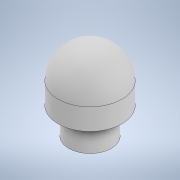
# Autodesk Inventor part: head
Saved by Autodesk Inventor 2022 (Build 260153000, 153)
## iProperties
Created: 2023-01-18
Part Number: head
Material: Generic
Document SubType Name: Modeling
Designer: zhong
Density: 1 g/cm^3
Appearance: Default
Author: zhong
Autodesk Inventor part; units mm, degrees
ref_plane "YZ Plane" through (0, 0, 0) normal (1, 0, 0) x (0, 1, 0)
ref_plane "XZ Plane" through (0, 0, 0) normal (0, 1, 0) x (-1, 0, 0)
ref_plane "XY Plane" through (0, 0, 0) normal (0, 0, 1) x (1, 0, 0)
sketch "Sketch1" plane through (0, 0, 0) normal (1, 0, 0) x (0, 1, 0)
  line L0 (0, 6) -> (4, 6)
  line L1 (0, -6) -> (4, -6)
  arc A0 (4, -6) -> (4, 6) centre (4, 0) ccw
  line L2 (0, 6) -> (0, 4)
  line L3 (0, 4) -> (-5, 4)
  line L4 (0, -6) -> (0, -4)
  line L5 (0, -4) -> (-5, -4)
  arc A1 (4, -4) -> (4, 4) centre (4, 0) ccw
  line L6 (2, 4) -> (4, 4)
  line L7 (2, -4) -> (4, -4)
  line L8 (2, -4) -> (2, -3)
  line L9 (2, -3) -> (-5, -3)
  line L10 (2, 4) -> (2, 3)
  line L11 (2, 3) -> (-5, 3)
  line L12 (-5, 4) -> (-5, 3)
  line L13 (-5, -3) -> (-5, -4)
  line L14 (-5, 0) -> (10, 0)
  point P0 (0, 0)
  point P1 (8, 0)
  dimension "d0" = 4
  dimension "d1" = 2
  dimension "d2" = 5
  dimension "d3" = 2
  dimension "d4" = 1
  dimension "d5" = 1
  constraints: 30 end point, 5 perpendicular, 5 point on circle, 5 vertical, 2 centre point, 2 horizontal, 2 tangent, 1 coincident
  measures "d0" distance of L0.start L0.end
  measures "d1" distance of L0.start L2.end
  measures "d2" distance of L2.end L3.end
  measures "d3" distance of L1.start L4.end
  measures "d4" distance of L7.start L8.end
  measures "d5" distance of L6.start L10.end
revolve "Revolution1" add sketch "Sketch1" angle 360 about axis through (0, -5, 0) along (0, 1, 0) contours A0 L1 L4 L5 L13 L9 L8 L7 A1 L14
body "Solid1"
